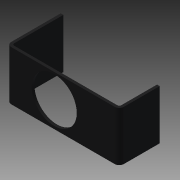
# Autodesk Inventor part: Beta_V2_BendFront01
Saved by Autodesk Inventor 2013 (Build 170138000, 138)
## iProperties
Created: 2015-02-17
Part Number: Beta_V2_BendFront01
Material: Aluminum 6061 Black Anodized
Document SubType Name: Modeling
Designer: spichelh
Density: 1 g/cm^3
Author: spichelh
Autodesk Inventor part; units mm, degrees
ref_plane "YZ Plane" through (0, 0, 0) normal (1, 0, 0) x (0, 1, 0)
ref_plane "XZ Plane" through (0, 0, 0) normal (0, 1, 0) x (-1, 0, 0)
ref_plane "XY Plane" through (0, 0, 0) normal (0, 0, 1) x (1, 0, 0)
sketch "Sketch3" plane through (0, 0, 0) normal (0, 1, 0) x (-1, 0, 0)
  line L0 (-57.5, 0) -> (57.5, 0)
  line L1 (62.5, -5) -> (62.5, -60)
  line L2 (-62.5, -45) -> (-62.5, -5)
  arc A0 (-57.5, 0) -> (-62.5, -5) centre (-57.5, -5) ccw
  arc A1 (62.5, -5) -> (57.5, 0) centre (57.5, -5) ccw
  line L3 (59.5, -60) -> (59.5, -5)
  arc A2 (59.5, -5) -> (57.5, -3) centre (57.5, -5) ccw
  line L4 (57.5, -3) -> (-57.5, -3)
  arc A3 (-57.5, -3) -> (-59.5, -5) centre (-57.5, -5) ccw
  line L5 (-59.5, -5) -> (-59.5, -45)
  line L6 (-62.5, -45) -> (-59.5, -45)
  line L7 (59.5, -60) -> (62.5, -60)
  point P0 (0, 0)
  point P1 (0, 0)
  dimension "d8" = 5
  dimension "d9" = 125
  dimension "d11" = 3
  dimension "d12" = 40
  dimension "d22" = 55
  constraints: 16 end point, 8 point on circle, 4 centre point, 4 tangent, 3 parallel, 3 perpendicular, 1 coincident, 1 equal radius, 1 horizontal, 1 midpoint, 4 other
  measures "d8" radius of A0
  measures "d9" distance between parallel lines of L1 L2
  measures "d11" distance between parallel lines of L0 L4
  measures "d12" distance of L2.start L2.end
  measures "d22" distance of L1.start L1.end
extrude "Extrusion3" add sketch "Sketch3" along normal blind 55
sketch "Sketch4" plane through (-57.5, 0, 0) normal (0, 0, 1) x (1, 0, 0)
  line L0 (0, 0) -> (115, 0) projected
  circle A0 centre (47.8, 28) radius 25
  line L1 (120, 0) -> (120, 55) projected
  line L2 (-5, 0) -> (-5, 55) projected
  point P0 (57.5, 0)
  dimension "d15" = 50
  dimension "d17" = 28
  dimension "d21" = 52.8
  constraints: 1 centre point
  measures "d15" diameter of A0
  measures "d17" distance from line of L0 A0.centre
  measures "d21" distance from line of L2 A0.centre
extrude "Extrusion4" cut sketch "Sketch4" against normal blind 60
body "Solid2"
